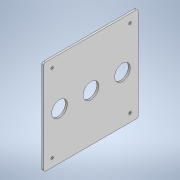
# Autodesk Inventor part: Bottom Plate
Saved by Autodesk Inventor 2022 (Build 260153000, 153)
## iProperties
Created: 2022-03-14
Part Number: Bottom Plate
Material: Generic
Document SubType Name: Modeling
Designer: ultra
Density: 1 g/cm^3
Appearance: Default
Author: ultra
Autodesk Inventor part; units mm, degrees
ref_plane "YZ Plane" through (0, 0, 0) normal (1, 0, 0) x (0, 1, 0)
ref_plane "XZ Plane" through (0, 0, 0) normal (0, 1, 0) x (-1, 0, 0)
ref_plane "XY Plane" through (0, 0, 0) normal (0, 0, 1) x (1, 0, 0)
sketch "Sketch1" plane through (0, 0, 0) normal (1, 0, 0) x (0, 1, 0)
  line L0 (-76.2, 76.2) -> (76.2, 76.2)
  line L1 (76.2, 76.2) -> (76.2, -76.2)
  line L2 (76.2, -76.2) -> (-76.2, -76.2)
  line L3 (-76.2, -76.2) -> (-76.2, 76.2)
  circle A0 centre (62.8611, 62.86) radius 2.032
  circle A1 centre (-62.8625, -62.8636) radius 2.032
  circle A2 centre (-0.0007, -88.9018) radius 2.032
  circle A3 centre (-62.8625, 62.86) radius 2.032
  circle A4 centre (88.8993, -0.0018) radius 2.032
  circle A5 centre (-88.9007, -0.0018) radius 2.032
  circle A6 centre (62.8611, -62.8636) radius 2.032
  circle A7 centre (-0.0007, 88.8982) radius 2.032
  circle A8 centre (-0.0007, -0.0018) radius 6.35
  dimension "d0" = 152.4
  dimension "d1" = 152.4
  dimension "d5" = 12.7
  constraints: 9 centre point, 8 end point, 2 parallel, 1 horizontal, 1 perpendicular
  measures "d0" distance of L1.end L2.end
  measures "d1" distance of L0.end L1.end
  measures "d5" diameter of A8
extrude "Extrusion2" add sketch "Sketch1" along normal blind 3.175 contours L0 L1 L2 L3 | A8
fillet "Fillet2" radius 3.175 4 edges at (1.5875, 76.2, 76.2) (1.5875, 76.2, -76.2) (1.5875, -76.2, 76.2) (1.5875, -76.2, -76.2)
sketch "Sketch2" plane through (3.175, 0, 0) normal (1, 0, 0) x (0, 0, -1)
  line L0 (-50.8, -50.8) -> (50.8, -50.8)
  line L1 (50.8, -50.8) -> (50.8, 50.8)
  line L2 (50.8, 50.8) -> (-50.8, 50.8)
  line L3 (-50.8, 50.8) -> (-50.8, -50.8)
  line L4 (-50.8, -50.8) -> (50.8, 50.8) construction
  line L5 (50.8, -50.8) -> (-50.8, 50.8) construction
  circle A0 centre (0, 0) radius 12.7
  line L6 (-12.7, 0) -> (-50.8, 38.1)
  line L7 (0, 12.7) -> (-38.1, 50.8)
  line L8 (-38.1, 50.8) -> (0, 12.7)
  line L9 (38.1, 50.8) -> (0, 12.7)
  line L10 (12.7, 0) -> (50.8, 38.1)
  line L11 (12.7, 0) -> (50.8, -38.1)
  line L12 (0, -12.7) -> (38.1, -50.8)
  line L13 (0, -12.7) -> (-38.1, -50.8)
  line L14 (-12.7, 0) -> (-50.8, -38.1)
  dimension "d9" = 101.6
  dimension "d10" = 101.6
  dimension "d11" = 25.4
  constraints: 30 end point, 10 point on line, 5 parallel, 4 point on circle, 2 midpoint, 2 perpendicular, 1 centre point, 1 coincident, 1 collinear, 1 horizontal
  measures "d9" distance of L2.end L1.end
  measures "d10" distance of L1.end L0.end
  measures "d11" diameter of A0
extrude "Extrusion3" [suppressed]
fillet "Fillet3" [suppressed]
sketch "Sketch4" plane through (0, 0, 0) normal (-1, 0, 0) x (0, 0, 1)
  circle A0 centre (0, 0) radius 12.7
  circle A1 centre (50.8, 0) radius 12.7
  circle A2 centre (-50.8, 0) radius 12.7
  dimension "d18" = 25.4
  dimension "d21" = 25.4
  dimension "d22" = 25.4
  dimension "d23" = 50.8
  dimension "d24" = 50.8
  constraints: 3 centre point, 1 coincident
  measures "d18" diameter of A0
  measures "d21" diameter of A1
  measures "d22" diameter of A2
  measures "d23" distance of A1.centre point (0, 0)
  measures "d24" distance of A2.centre point (0, 0)
extrude "Extrusion6" cut sketch "Sketch4" against normal blind 25.4
body "Solid2"
